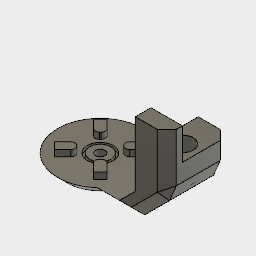
Foot Cross (Autodesk Fusion 360 design; units mm, degrees)
Autodesk Fusion 360 part; units mm, degrees
note: some values were not read from the file. Set by a fixed rule: which sketch regions a step uses.
sketch "Sketch1" plane through (0, 0, 0) normal (0, 1, 0) x (1, 0, 0)
  circle A0 centre (0, 0) radius 13.5
  line L0 (9.0692, -10) -> (9.0692, 10)
  line L1 (9.0692, 10) -> (21.0692, 10)
  line L2 (21.0692, 10) -> (21.0692, -10)
  line L3 (21.0692, -10) -> (9.0692, -10)
  line L4 (9.0692, -10) -> (9.0692, 10)
  dimension "d1" = 27
  dimension "d4" = 20
  dimension "d5" = 12
  dimension "d6" = 20
  measures "d1" diameter of A0
  measures "d4" distance of L0.start L0.end
  measures "d5" distance of L0.end L1.end
  measures "d6" distance of L0.end L0.start
extrude "Extrude1" add sketch "Sketch1" along normal blind 3
sketch "Sketch2" plane through (0, 3, 0) normal (0, 1, 0) x (-1, 0, 0)
  arc A0 (-9.0692, -10) -> (-9.0692, 10) centre (0, 0) ccw
  line L0 (-9.0692, 10) -> (-21.0692, 10)
  line L1 (-21.0692, 10) -> (-21.0692, -10)
  line L2 (-21.0692, -10) -> (-9.0692, -10)
  circle A1 centre (0, 0) radius 1.5
  dimension "d11" = 3
  measures "d11" diameter of A1
extrude "Extrude2" cut sketch "Sketch2" against normal blind 7 contours A1
sketch "Sketch3" plane through (0, 3, 0) normal (0, 1, 0) x (-1, 0, 0)
  circle A0 centre (0, 0) radius 1.5
  arc A1 (-9.0692, -10) -> (-9.0692, 10) centre (0, 0) ccw
  line L0 (-9.0692, 10) -> (-21.0692, 10)
  line L1 (-21.0692, 10) -> (-21.0692, -10)
  line L2 (-21.0692, -10) -> (-9.0692, -10)
  line L3 (0, 0) -> (7.2478, -7.2478) construction
  line L4 (0, 0) -> (-7.2478, 7.2478) construction
  line L5 (0, 0) -> (7.2478, 7.2478) construction
  line L6 (0, 0) -> (10.5, 0) construction
  line L7 (0, 0) -> (-7.2478, -7.2478) construction
  line L8 (-7.2478, 7.2478) -> (-6.1872, 8.3085) construction
  line L9 (7.2478, 7.2478) -> (8.3085, 6.1872) construction
  line L10 (7.2478, -7.2478) -> (6.1872, -8.3085) construction
  line L11 (-7.2478, -7.2478) -> (-8.3085, -6.1872) construction
  line L12 (-8.3085, -6.1872) -> (-4.773, -2.6517)
  line L13 (-4.773, -2.6517) -> (-2.6517, -4.773)
  line L14 (-4.773, -2.6517) -> (-1.773, -2.6517) construction
  line L15 (-2.6517, -4.773) -> (-6.1872, -8.3085)
  line L16 (-6.1872, -8.3085) -> (-8.3085, -6.1872)
  line L17 (-6.1872, 8.3085) -> (-8.3085, 6.1872)
  line L18 (-8.3085, 6.1872) -> (-4.773, 2.6517)
  line L19 (-4.773, 2.6517) -> (-2.6517, 4.773)
  line L20 (-4.773, 2.6517) -> (-1.773, 2.6517) construction
  line L21 (-2.6517, 4.773) -> (-6.1872, 8.3085)
  line L22 (8.3085, 6.1872) -> (6.1872, 8.3085)
  line L23 (6.1872, 8.3085) -> (2.6517, 4.773)
  line L24 (6.1872, 8.3085) -> (11.1872, 8.3085) construction
  line L25 (2.6517, 4.773) -> (4.773, 2.6517)
  line L26 (4.773, 2.6517) -> (8.3085, 6.1872)
  line L27 (6.1872, -8.3085) -> (8.3085, -6.1872)
  line L28 (8.3085, -6.1872) -> (4.773, -2.6517)
  line L29 (4.773, -2.6517) -> (2.6517, -4.773)
  line L30 (2.6517, -4.773) -> (6.1872, -8.3085)
  dimension "d15" = 10.25
  dimension "d16" = 10.25
  dimension "d18" = 45
  dimension "d19" = 10.25
  dimension "d20" = 10.25
  dimension "d79" = 1.5
  dimension "d80" = 1.5
  dimension "d81" = 1.5
  dimension "d84" = 1.5
  dimension "d85" = 5
  dimension "d86" = 45
  dimension "d87" = 3
  dimension "d88" = 5
  dimension "d89" = 3
  dimension "d90" = 5
  dimension "d91" = 45
  dimension "d92" = 3
  dimension "d93" = 3
  dimension "d94" = 135
  dimension "d95" = 5
  dimension "d96" = 3
  dimension "d97" = 3
  dimension "d98" = 5
  dimension "d99" = 3
  measures "d15" distance of A0.centre L3.end
  measures "d16" distance of A0.centre L4.end
  measures "d18" angle of L5 L6
  measures "d19" distance of A0.centre L5.end
  measures "d20" distance of A0.centre L7.end
  measures "d79" distance of L4.end L8.end
  measures "d80" distance of L5.end L9.end
  measures "d81" distance of L3.end L10.end
  measures "d84" distance of L7.end L11.end
  measures "d85" distance of L11.end L12.end
  measures "d86" angle of L13 L14
  measures "d87" distance of L12.end L13.end
  measures "d88" distance of L13.end L15.end
  measures "d89" distance of L8.end L17.end
  measures "d90" distance of L17.end L18.end
  measures "d91" angle of L19 L20
  measures "d92" distance of L18.end L19.end
  measures "d93" distance of L9.end L22.end
  measures "d94" angle of L23 L24
  measures "d95" distance of L22.end L23.end
  measures "d96" distance of L23.end L25.end
  measures "d97" distance of L10.end L27.end
  measures "d98" distance of L27.end L28.end
  measures "d99" distance of L28.end L29.end
extrude "Extrude12" add sketch "Sketch3" along normal blind 2 contours L12 L13 L15 L16 | L17 L18 L19 L21 | L22 L23 L25 L26 | L27 L28 L29 L30
sketch "Sketch4" plane through (0, 3, 0) normal (0, 1, 0) x (-1, 0, 0)
  circle A0 centre (0, 0) radius 1.5
  arc A1 (-9.0692, -10) -> (-9.0692, 10) centre (0, 0) ccw
  line L0 (-9.0692, 10) -> (-21.0692, 10)
  line L1 (-21.0692, 10) -> (-21.0692, -10)
  line L2 (-21.0692, -10) -> (-9.0692, -10)
  circle A2 centre (0, 0) radius 3.4
  circle A3 centre (0, 0) radius 4.125
  line L3 (-2.6517, 4.773) -> (-4.773, 2.6517)
  line L4 (-4.773, 2.6517) -> (-8.3085, 6.1872)
  line L5 (-8.3085, 6.1872) -> (-6.1872, 8.3085)
  line L6 (-6.1872, 8.3085) -> (-2.6517, 4.773)
  line L7 (4.773, 2.6517) -> (2.6517, 4.773)
  line L8 (2.6517, 4.773) -> (6.1872, 8.3085)
  line L9 (6.1872, 8.3085) -> (8.3085, 6.1872)
  line L10 (8.3085, 6.1872) -> (4.773, 2.6517)
  line L11 (-6.1872, -8.3085) -> (-8.3085, -6.1872)
  line L12 (-8.3085, -6.1872) -> (-4.773, -2.6517)
  line L13 (-4.773, -2.6517) -> (-2.6517, -4.773)
  line L14 (-2.6517, -4.773) -> (-6.1872, -8.3085)
  line L15 (2.6517, -4.773) -> (4.773, -2.6517)
  line L16 (4.773, -2.6517) -> (8.3085, -6.1872)
  line L17 (8.3085, -6.1872) -> (6.1872, -8.3085)
  line L18 (6.1872, -8.3085) -> (2.6517, -4.773)
  dimension "d42" = 6.8
  dimension "d43" = 8.25
  measures "d42" diameter of A2
  measures "d43" diameter of A3
extrude "Extrude4" cut sketch "Sketch4" against normal blind 1 contours A3
sketch "Sketch5" plane through (0, 3, 0) normal (0, 1, 0) x (-1, 0, 0)
  arc A0 (-9.0692, -10) -> (-9.0692, 10) centre (0, 0) ccw
  line L0 (-9.0692, 10) -> (-21.0692, 10)
  line L1 (-21.0692, 10) -> (-21.0692, -10)
  line L2 (-21.0692, -10) -> (-9.0692, -10)
  circle A1 centre (0, 0) radius 4.125
  line L3 (-21.0692, -10) -> (-31.0692, -10)
  line L4 (-31.0692, -10) -> (-31.0692, 10)
  line L5 (-31.0692, 10) -> (-21.0692, 10)
  line L6 (-21.0692, 10) -> (-21.0692, -10)
  line L7 (2.6517, -4.773) -> (4.773, -2.6517)
  line L8 (4.773, -2.6517) -> (8.3085, -6.1872)
  line L9 (8.3085, -6.1872) -> (6.1872, -8.3085)
  line L10 (6.1872, -8.3085) -> (2.6517, -4.773)
  line L11 (-6.1872, -8.3085) -> (-8.3085, -6.1872)
  line L12 (-8.3085, -6.1872) -> (-4.773, -2.6517)
  line L13 (-4.773, -2.6517) -> (-2.6517, -4.773)
  line L14 (-2.6517, -4.773) -> (-6.1872, -8.3085)
  line L15 (4.773, 2.6517) -> (2.6517, 4.773)
  line L16 (2.6517, 4.773) -> (6.1872, 8.3085)
  line L17 (6.1872, 8.3085) -> (8.3085, 6.1872)
  line L18 (8.3085, 6.1872) -> (4.773, 2.6517)
  line L19 (-2.6517, 4.773) -> (-4.773, 2.6517)
  line L20 (-4.773, 2.6517) -> (-8.3085, 6.1872)
  line L21 (-8.3085, 6.1872) -> (-6.1872, 8.3085)
  line L22 (-6.1872, 8.3085) -> (-2.6517, 4.773)
  dimension "d46" = 10
  dimension "d47" = 20
  measures "d46" distance of L1.end L3.end
  measures "d47" distance of L1.end L0.end
extrude "Extrude5" add sketch "Sketch5" along normal blind 16.5 contours L1 L3 L4 L5 L6
sketch "Sketch6" plane through (0, 19.5, 0) normal (0, 1, 0) x (-1, 0, 0)
  line L0 (-21.0692, 10) -> (-31.0692, 10)
  line L1 (-31.0692, 10) -> (-31.0692, -10)
  line L2 (-31.0692, -10) -> (-21.0692, -10)
  line L3 (-21.0692, -10) -> (-21.0692, 10)
  line L4 (-21.0692, 10) -> (-31.0692, 10)
  line L5 (-31.0692, 10) -> (-31.0692, 5)
  line L6 (-31.0692, 5) -> (-21.0692, 5)
  line L7 (-21.0692, 5) -> (-21.0692, 10)
  dimension "d50" = 10
  dimension "d51" = 5
  measures "d50" distance of L0.start L0.end
  measures "d51" distance of L0.start L6.end
extrude "Extrude6" add sketch "Sketch6" along normal blind 10 contours L0 L1 L3 L4 L5 L6 L7
sketch "Sketch7" plane through (0, 19.5, 0) normal (0, 1, 0) x (-1, 0, 0)
  line L0 (-21.0692, 5) -> (-31.0692, 5)
  line L1 (-31.0692, 5) -> (-31.0692, -10)
  line L2 (-31.0692, -10) -> (-21.0692, -10)
  line L3 (-21.0692, -10) -> (-21.0692, 5)
  line L4 (-21.0692, -10) -> (-21.0692, 10)
  line L5 (-21.0692, 0) -> (-26.0692, 0)
  circle A0 centre (-26.0692, 0) radius 3.4
  dimension "d54" = 5
  dimension "d55" = 6.8
  measures "d54" distance of L5.start L5.end
  measures "d55" diameter of A0
extrude "Extrude7" cut sketch "Sketch7" against normal blind 9 contours A0
sketch "Sketch8" plane through (0, 10.5, 0) normal (0, 1, 0) x (-1, 0, 0)
  circle A0 centre (-26.0692, 0) radius 3.4
  circle A1 centre (-26.0692, 0) radius 1.75
  dimension "d60" = 3.5
  measures "d60" diameter of A1
sketch "Sketch9" plane through (0, 0, 10) normal (0, 0, 1) x (1, 0, 0)
  line L0 (9.0692, 0) -> (21.0692, 0)
  line L1 (21.0692, 0) -> (21.0692, 3)
  line L2 (21.0692, 3) -> (9.0692, 3)
  line L3 (9.0692, 3) -> (9.0692, 0)
  line L4 (21.0692, 0) -> (27.5513, 6.4821)
  line L5 (21.0692, 0) -> (30.2363, 0) construction
  line L6 (21.0692, 0) -> (21.0692, 3)
  line L7 (31.0692, 3) -> (21.0692, 3)
  line L8 (21.0692, 3) -> (26.0692, 3)
  dimension "d61" = 45
  measures "d61" angle of L4 L5
extrude "Extrude8" add sketch "Sketch9" against normal blind 20 contours L1 L4 L6 L7 L8
sketch "Sketch10" plane through (0, 0, 10) normal (0, 0, 1) x (1, 0, 0)
  line L0 (24.0692, 3) -> (31.0692, 3)
  line L1 (31.0692, 3) -> (31.0692, 29.5)
  line L2 (31.0692, 29.5) -> (21.0692, 29.5)
  line L3 (21.0692, 29.5) -> (21.0692, 3)
  line L4 (21.0692, 3) -> (9.0692, 3)
  line L5 (9.0692, 3) -> (9.0692, 0)
  line L6 (9.0692, 0) -> (21.0692, 0)
  line L7 (21.0692, 0) -> (24.0692, 3)
  line L8 (24.0692, 3) -> (32.4914, 11.4222)
  line L9 (24.0692, 3) -> (35.98, 3) construction
  dimension "d64" = 45
  measures "d64" angle of L8 L9
extrude "Extrude9" cut sketch "Sketch10" against normal blind 77 contours L0 L1 L8
extrude "Extrude10" cut sketch "Sketch8" against normal blind 20 contours A1
ref_plane "WorkPlane1" through (26.0692, 7.5, 0) normal (0, 1, 0) x (-1, 0, 0)
sketch "Sketch11" plane through (26.0692, 7.5, 0) normal (0, 1, 0) x (1, 0, 0)
  circle A0 centre (0, 0) radius 3
  dimension "d70" = 6
  measures "d70" diameter of A0
extrude "Extrude11" cut sketch "Sketch11" against normal blind 10
chamfer "Chamfer1" distance 3 angle 45 3 edges at (15.0692, 0, 10) (-13.5, 0, 0) (15.0692, 0, -10)
chamfer "Chamfer2" distance 5 angle 45 1 edges at (21.0692, 3, 0)
chamfer "Chamfer3" distance 3 angle 45 5 edges at (27.5692, 6.5, 10) (31.0692, 19.75, 10) (27.5692, 6.5, -10) (31.0692, 14.75, -10) (31.0692, 10, 0)
fillet "Fillet2" radius 1.35 8 edges at (-2.6517, 4, 4.773) (-4.773, 4, 2.6517) (-4.773, 4, -2.6517) (-2.6517, 4, -4.773) (2.6517, 4, -4.773) (4.773, 4, -2.6517) (4.773, 4, 2.6517) (2.6517, 4, 4.773)
extrude "Extrude13" cut 1 faces at (26.7358, 29.5, 6.6667) along direction (0, -1, 0) blind 1
extrude "Extrude14" cut 1 faces at (24.817, 19.5, -7.7716) along direction (0, -1, 0) blind 1
extrude "Extrude15" cut 1 faces at (23.2318, 10.5, -0.1689) along direction (0, -1, 0) blind 1
equation "d5 = KneeSeparation"
equation "d7 = BottomThickness"
equation "BottomThickness = 3 mm"
equation "KneeSeparation = 12 mm"
equation "d11 = ServoScrewHole"
equation "ScrewHole = 3.0 mm"
equation "HornFit = 1.35 mm"
equation "d54 = HolePosX"
equation "d55 = HoleSize"
equation "HolePosX = 5 mm"
equation "HoleSize = 6.8 mm"
equation "d58 = -HoleDepth"
equation "d60 = SpacerScrewHole"
equation "d70 = HoleFit"
equation "HoleFit = 6 mm"
equation "ChamferStrength = 5 mm"
equation "Chamfer3 = 3 mm"
equation "d76 = Chamfer3"
equation "d77 = ChamferStrength"
equation "d78 = Chamfer3"
equation "FilletFIT = 1.35 mm"
equation "d103 = FilletFIT"
equation "HoleDepth = 9 mm"
equation "ServoScrewHole = 3 mm"
equation "SpacerScrewHole = 3.5 mm"
